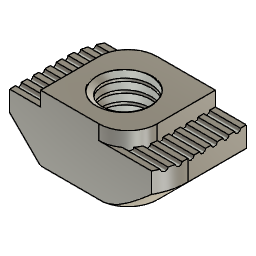
JAL- M4 T-Nut for 2020 extrusion (Autodesk Fusion 360 design; units mm, degrees)
Autodesk Fusion 360 part; units mm, degrees
sketch "Central profile" plane through (0, 0, 0) normal (0, 0, 1) x (1, 0, 0) in component "M4 T-Nut for 2020 extrusion"
  line L0 (3, 3) -> (-1, 3)
  line L1 (-3, 1) -> (-3, -3)
  line L2 (-3, -3) -> (1, -3)
  line L3 (3, -1) -> (3, 3)
  line L4 (3, 3) -> (-3, -3) construction
  line L5 (-3, 3) -> (3, -3) construction
  arc A0 (-1, 3) -> (-3, 1) centre (-1, 1) ccw
  arc A1 (1, -3) -> (3, -1) centre (1, -1) ccw
  circle A2 centre (0, 0) radius 2
  dimension "d1" = 6
  dimension "d2" = 6
  dimension "d3" = 2
  dimension "d4" = 4
  constraint horizontal L0
  constraint perpendicular L0 L1
  constraint parallel L0 L2
  constraint parallel L1 L3
  constraint coincident L4 A2.centre
  constraint coincident L5 A2.centre
  constraint coincident A2.centre origin
  constraint coincident L5.start L0
  constraint coincident L5.start L1
  constraint tangent L0 A0
  constraint tangent L1 A0
  constraint coincident L5.end L3
  constraint coincident L5.end L2
  constraint tangent L3 A1
  constraint tangent L2 A1
  constraint equal A0 A1
  measures "d1" distance of L1.end L5.end
  measures "d2" distance of L5.start L1.end
  measures "d3" radius of A0
  measures "d4" diameter of A2
extrude "Extrude1" add sketch "Central profile" along normal blind 4.5 in component "M4 T-Nut for 2020 extrusion"
sketch "Protrusion profile" plane through (0, 0, 0) normal (0, 0, 1) x (1, 0, 0) in component "M4 T-Nut for 2020 extrusion"
  circle A0 centre (0, 0) radius 2 construction
  arc A1 (1, -3) -> (3, -1) centre (1, -1) ccw construction
  line L0 (3, -1) -> (3, 3) construction
  line L1 (3, 3) -> (-1, 3) construction
  arc A2 (-1, 3) -> (-3, 1) centre (-1, 1) ccw construction
  line L2 (-3, 1) -> (-3, -3) construction
  line L3 (-3, -3) -> (1, -3) construction
  line L4 (5.125, 5.125) -> (-1, 5.125) construction
  arc A3 (-1, 5.125) -> (-5.125, 1) centre (-1, 1) ccw
  line L5 (-5.125, 1) -> (-5.125, -5.125)
  line L6 (-5.125, -5.125) -> (1, -5.125) construction
  arc A4 (1, -5.125) -> (5.125, -1) centre (1, -1) ccw
  line L7 (5.125, -1) -> (5.125, 5.125)
  line L8 (-4.6077, 3) -> (5.125, 3)
  line L9 (-5.125, -3) -> (4.6077, -3)
  circle A5 centre (0, 0) radius 2
  dimension "d7" = 2.125
  constraint coincident A3 L8.start
  constraint coincident L7 L8.end
  constraint collinear L1 L8
  constraint coincident L5 L9.start
  constraint coincident A4 L9.end
  constraint collinear L3 L9
  constraint concentric A0 A5
extrude "Extrude2" add sketch "Protrusion profile" along normal up to surface (3.5 mm away) in component "M4 T-Nut for 2020 extrusion"
chamfer "Chamfer1" distance 2.1 angle 45 4 edges at (-4.9936, 2.0329, 0) (-5.125, -1, 0) (4.9936, -2.0329, 0) (5.125, 1, 0) in component "M4 T-Nut for 2020 extrusion"
extrude "Extrude3" cut 1 faces at (-2.637, -0.8632, 4.5) along direction (0, 0, -1) blind 1.5 in component "M4 T-Nut for 2020 extrusion"
sketch "Grip cutting profile" plane through (0, 0, 0) normal (1, 0, 0) x (0, 1, 0) in component "M4 T-Nut for 2020 extrusion"
  line L0 (-1, 3.5) -> (-3, 3.5) construction
  line L1 (-3, 3.5) -> (-1, 3.5) construction
  line L2 (-1, 3.5) -> (3, 3.5) construction
  line L3 (3, 3.5) -> (-1, 3.5) construction
  circle A0 centre (-2.4, 3.5) radius 0.2
  circle A1 centre (-1.6, 3.5) radius 0.2
  circle A2 centre (-0.8, 3.5) radius 0.2
  circle A3 centre (0, 3.5) radius 0.2
  circle A4 centre (0.8, 3.5) radius 0.2
  circle A5 centre (1.6, 3.5) radius 0.2
  circle A6 centre (2.4, 3.5) radius 0.2
  dimension "d14" = 0.4
  dimension "d17" = -0.8
  dimension "d18" = 0
  dimension "d19" = 0.6
  dimension "d20" = 0.6
  measures "d14" diameter of A0
  measures "d19" distance of L0.end A0.centre
  measures "d20" distance of L2.end A6.centre
extrude "Extrude4" cut sketch "Grip cutting profile" along normal through all and the other way through all in component "M4 T-Nut for 2020 extrusion"
extrude "Extrude5" add 1 faces at (-2.637, -0.8632, 3) along direction (0, 0, 1) blind 1.5 in component "M4 T-Nut for 2020 extrusion"
thread "Thread1" "ISO Metric profile 4.0 M4x0.7 6H" major diameter 4.1095 minor diameter 3.332 pitch 0.7 angle 60 modelled right hand crest width 0.193 on face at (1.9975, -0.0997, 3) crest through (1.666, 0, 0.175) in component "M4 T-Nut for 2020 extrusion"
component "M4 T-Nut for 2020 extrusion" placed x (1, 0, 0) y (0, 1, 0) z (0, 0, 1) at (0, 0, 0)
equation "d19 = d14 / 2 + d14"
named bodies: "M4 t-Nut"
